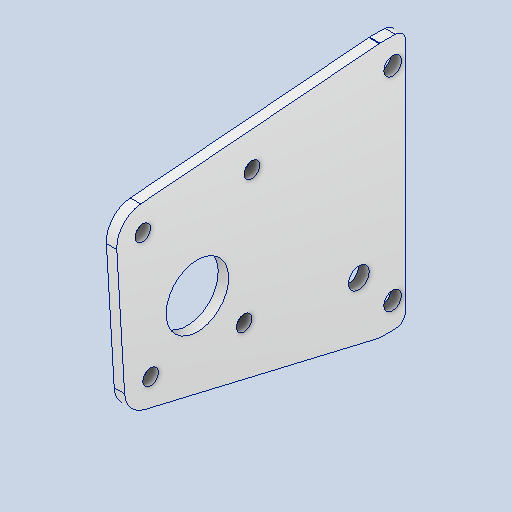
# Autodesk Inventor part: install-encoder-v1-Plate-E-F
Saved by Autodesk Inventor 2024 (Build 280153000, 153)
## iProperties
Created: 2024-02-12
Part Number: install-encoder-v1-Plate-E-F
Material: アルミニウム 6061
Document SubType Name: Modeling
Designer: haruy
Density: 2.7 g/cm^3
Appearance: アルミニウム - フラット
Author: haruy
Autodesk Inventor part; units mm, degrees
ref_plane "YZ Plane" through (0, 0, 0) normal (1, 0, 0) x (0, 1, 0)
ref_plane "XZ Plane" through (0, 0, 0) normal (0, 1, 0) x (-1, 0, 0)
ref_plane "XY Plane" through (0, 0, 0) normal (0, 0, 1) x (1, 0, 0)
derived "install-encoder-v1-Sketch-Base.ipt"
sketch "横から" plane through (0, 0, 0) normal (1, 0, 0) x (0, 1, 0)
  circle A0 centre (0, 0) radius 30
  circle A1 centre (-12.5, -31) radius 2
  circle A2 centre (57.5, -31) radius 2
  line L0 (28.047, 14.387) -> (-15.329, 14.387)
  line L1 (-15.329, 14.387) -> (-15.329, -14.388)
  line L2 (-15.329, -14.388) -> (28.047, -14.388)
  line L3 (28.047, -14.388) -> (28.047, 14.387)
  circle A3 centre (15.748, -10.478) radius 1.5
  circle A4 centre (-8.98, -8.98) radius 1.5
  line L4 (-15.329, -0.0005) -> (28.047, -0.0005)
  circle A5 centre (15.748, 10.477) radius 1.5
  circle A6 centre (-8.98, 8.979) radius 1.5
  circle A7 centre (0, 0) radius 6
  line L5 (14.5, -40) -> (-14.5, -40)
  line L6 (-14.5, -40) -> (-14.5, -44.5)
  line L7 (-14.5, -44.5) -> (14.5, -44.5)
  line L8 (14.5, -44.5) -> (14.5, -40)
  line L9 (40.5, -44.5) -> (-14.5, -44.5)
  line L10 (-14.5, -44.5) -> (-14.5, -50)
  line L11 (-14.5, -50) -> (40.5, -50)
  line L12 (40.5, -50) -> (40.5, -44.5)
  line L13 (-24.5, -40) -> (24.5, -40)
  line L14 (24.5, -40) -> (24.5, -35)
  line L15 (24.5, -35) -> (-24.5, -35)
  line L16 (-24.5, -35) -> (-24.5, -40)
  circle A8 centre (-19.5, -37.5) radius 1.7
  circle A9 centre (19.5, -37.5) radius 1.7
  circle A10 centre (15.748, 10.477) radius 5
  circle A11 centre (-8.98, 8.979) radius 5
  line L17 (24.5, -35) -> (20.7312, 10.8863)
  line L18 (15.4457, 15.4679) -> (-9.2823, 13.9699)
  line L19 (-13.8462, 10.1278) -> (-24.5, -35)
  circle A12 centre (0, 0) radius 10
  line L20 (24.5, -35) -> (9.307, 3.6578)
  line L21 (-24.5, -35) -> (-9.307, 3.6578)
  point P0 (-14.5, -40)
  point P1 (30, 0)
sketch "上から" plane through (0, 0, 0) normal (0, 0, 1) x (1, 0, 0)
  line L0 (-8.7169, 37.9045) -> (16.8831, 37.9045)
  line L1 (16.8831, 37.9045) -> (16.8831, -22.0955)
  line L2 (16.8831, -22.0955) -> (-8.7169, -22.0955)
  line L3 (-8.7169, -22.0955) -> (-8.7169, 37.9045)
  line L4 (16.8831, 29.5244) -> (20.6331, 29.5244)
  line L5 (20.6331, 29.5244) -> (20.6331, -7.4709)
  line L6 (20.6331, -7.4709) -> (16.8831, -7.4709)
  line L7 (16.8831, -7.4709) -> (16.8831, 29.5244)
  line L8 (23.6331, 14.9045) -> (27.1331, 14.9045)
  line L9 (27.1331, 14.9045) -> (27.1331, 0.9045)
  line L10 (27.1331, 0.9045) -> (23.6331, 0.9045)
  line L11 (23.6331, 0.9045) -> (23.6331, 14.9045)
  line L12 (24.4331, 14.9045) -> (24.4331, 0.9045)
  line L13 (-15.2169, 14.9045) -> (-11.7169, 14.9045)
  line L14 (-11.7169, 14.9045) -> (-11.7169, 0.9045)
  line L15 (-11.7169, 0.9045) -> (-15.2169, 0.9045)
  line L16 (-15.2169, 0.9045) -> (-15.2169, 14.9045)
  line L17 (-12.5169, 0.9045) -> (-12.5169, 14.9045)
  line L18 (-14.5169, 47.9045) -> (-12.5169, 47.9045)
  line L19 (-12.5169, 47.9045) -> (-12.5169, -25.1723)
  line L20 (-12.5169, -25.1723) -> (-14.5169, -25.1723)
  line L21 (-14.5169, -25.1723) -> (-14.5169, 47.9045)
  line L22 (24.4331, 47.768) -> (26.4331, 47.768)
  line L23 (26.4331, 47.768) -> (26.4331, -21.9286)
  line L24 (26.4331, -21.9286) -> (24.4331, -21.9286)
  line L25 (24.4331, -21.9286) -> (24.4331, 47.768)
  circle A0 centre (36.9331, 38.9045) radius 8.5
  line L26 (-5.9169, 47.9045) -> (14.0831, 47.9045)
  line L27 (14.0831, 47.9045) -> (14.0831, 52.4045)
  line L28 (14.0831, 52.4045) -> (-5.9169, 52.4045)
  line L29 (-5.9169, 52.4045) -> (-5.9169, 47.9045)
  line L30 (-0.4169, 57.9045) -> (8.5831, 57.9045)
  line L31 (8.5831, 57.9045) -> (8.5831, 52.4045)
  line L32 (8.5831, 52.4045) -> (-0.4169, 52.4045)
  line L33 (-0.4169, 52.4045) -> (-0.4169, 57.9045)
  line L34 (-14.5169, 59.9045) -> (45.4331, 59.9045)
  line L35 (45.4331, 59.9045) -> (45.4331, 57.9045)
  line L36 (45.4331, 57.9045) -> (-14.5169, 57.9045)
  line L37 (-14.5169, 57.9045) -> (-14.5169, 59.9045)
  line L38 (26.4331, 22.292) -> (35.4331, 22.292)
  line L39 (35.4331, 22.292) -> (35.4331, -6.483)
  line L40 (35.4331, -6.483) -> (26.4331, -6.483)
  line L41 (26.4331, -6.483) -> (26.4331, 22.292)
  line L42 (-8.7169, 7.9045) -> (16.8831, 7.9045)
  line L43 (4.0831, 37.9045) -> (4.0831, -22.0955)
  line L44 (-12.5169, 47.9045) -> (24.4331, 47.9045)
  line L45 (24.4331, 47.9045) -> (24.4331, 42.9045)
  line L46 (24.4331, 42.9045) -> (-12.5169, 42.9045)
  line L47 (-12.5169, 42.9045) -> (-12.5169, 47.9045)
  line L48 (34.9331, 41.1503) -> (38.9331, 41.1503)
  line L49 (38.9331, 41.1503) -> (38.9331, 36.1752)
  line L50 (38.9331, 36.1752) -> (34.9331, 36.1752)
  line L51 (34.9331, 36.1752) -> (34.9331, 41.1503)
  point P0 (0, 0)
sketch "後ろから" plane through (0, 0, 0) normal (0, 1, 0) x (-1, 0, 0)
  point P0 (0, 0)
extrude "押し出し1" add sketch "横から" along normal blind 2 contours L19 L1 L21 A0 | A0 L21 L19 | A10 L0 | L0 A10 | L17 L2 L20 A3 L4 | L4 L20 A12 A11 L18 L0 A10 L17 | L17 L20 A0 | A0 L20 L2 L17 | L21 L1 L2 L20 A0 | A0 L20 L15 L21 | L19 A11 A12 L21 L4 L1 | L15 L14 L13 L5 L16 | L0 L18 A10 | L20 A3 L2 L1 L21 L4 A12 | L4 A12 L20 | L1 L4 L21 | A11 A12 | A12 L4 A7 | L4 A7 A12 A11 | L21 A12 L4 | A12 A11
fillet "フィレット1" radius 2 4 edges at (1, 24.5, -40) (1, -24.5, -40) (1, 24.5, -35) (1, -24.5, -35)
